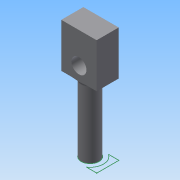
# Autodesk Inventor part: charniere
Saved by Autodesk Inventor 2015 (Build 190159000, 159)
## iProperties
Created: 2015-06-19
Part Number: charniere
Material: Générique
Document SubType Name: Modeling
Designer: Gregwar
Density: 1 g/cm^3
Appearance: Par défaut
Author: Gregwar
Autodesk Inventor part; units mm, degrees
ref_plane "YZ Plane" through (0, 0, 0) normal (1, 0, 0) x (0, 1, 0)
ref_plane "XZ Plane" through (0, 0, 0) normal (0, 1, 0) x (-1, 0, 0)
ref_plane "XY Plane" through (0, 0, 0) normal (0, 0, 1) x (1, 0, 0)
sketch "Esquisse7" plane through (0, 0, 0) normal (0, 1, 0) x (-1, 0, 0)
  line L0 (0, 0) -> (8, 0)
  line L1 (8, 0) -> (8, -10)
  line L2 (8, -10) -> (0, -10)
  line L3 (0, -10) -> (0, 0)
  line L4 (4, -10) -> (4, 0) construction
  circle A0 centre (4, -7) radius 1.7
  dimension "d15" = 3.4
  dimension "d16" = 10
  dimension "d17" = 8
  dimension "d24" = 3
  constraints: 10 end point, 2 midpoint, 2 parallel, 1 centre point, 1 horizontal, 1 perpendicular, 1 point on line
  measures "d15" diameter of A0
  measures "d16" distance of L2.end L0.start
  measures "d17" distance of L0.start L0.end
  measures "d24" distance from line of L2 A0.centre
extrude "Extrusion5" add sketch "Esquisse7" along normal blind 5
sketch "Esquisse8" plane through (0, 0, -10) normal (0, 0, -1) x (-1, 0, 0)
  line L0 (8, 5) -> (0, 5) construction
  line L1 (4, 5) -> (4, 0) construction
  line L2 (0, 0) -> (8, 0) construction
  circle A0 centre (4, 2.5) radius 2
  dimension "d20" = 4
  constraints: 3 midpoint, 2 end point, 1 centre point
  measures "d20" diameter of A0
extrude "Extrusion6" add sketch "Esquisse8" along normal blind 16
fillet "Congé3" radius 1 1 edges at (-2, 2.5, -10)
sketch "Esquisse9" plane through (-4, 2.5, -26) normal (0, 0, -1) x (-1, 0, 0)
  circle A0 centre (0, 0) radius 2 projected
  arc A1 (-1.6583, 2.5) -> (-1.6583, -2.5) centre (0, 0) ccw projected
  arc A2 (-1.6583, 2.5) -> (-1.6583, -2.5) centre (0, 0) ccw projected
  line L0 (-4, 2.5) -> (-1.6583, 2.5) projected
  line L1 (-4, -2.5) -> (-4, 2.5) projected
  line L2 (-1.6583, -2.5) -> (-4, -2.5) projected
  point P0 (-4, -2.5)
